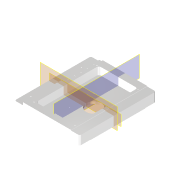
# Autodesk Inventor part: 00_xystage_gp-010b_base
Saved by Autodesk Inventor 2022 (Build 260153000, 153)
## iProperties
Created: 2022-06-02
Part Number: 00_xystage_gp-010b_base
Material: Generisch
Document SubType Name: Modellieren
Designer: diederichbenedict
Density: 1 g/cm^3
Appearance: Glatt - Weiß
Sheet Metal Rule: Standard_mm
Author: diederichbenedict
Autodesk Inventor part; units mm, degrees
ref_plane "YZ Plane" through (0, 0, 0) normal (1, 0, 0) x (0, 1, 0)
ref_plane "XZ Plane" through (0, 0, 0) normal (0, 1, 0) x (-1, 0, 0)
ref_plane "XY Plane" through (0, 0, 0) normal (0, 0, 1) x (1, 0, 0)
sketch "Skizze1" plane through (0, 0, 0) normal (0, 1, 0) x (-1, 0, 0)
  line L0 (76, -93.75) -> (-76, -93.75)
  line L1 (-80, -89.75) -> (-80, 89.75)
  line L2 (-76, 93.75) -> (76, 93.75)
  line L3 (80, 89.75) -> (80, -89.75)
  line L4 (80, -93.75) -> (-80, 93.75) construction
  line L5 (-80, -93.75) -> (80, 93.75) construction
  arc A0 (80, 89.75) -> (76, 93.75) centre (76, 89.75) ccw
  arc A1 (76, -93.75) -> (80, -89.75) centre (76, -89.75) ccw
  arc A2 (-80, -89.75) -> (-76, -93.75) centre (-76, -89.75) ccw
  arc A3 (-76, 93.75) -> (-80, 89.75) centre (-76, 89.75) ccw
  line L6 (43.7, 77.95) -> (-51.7, 77.95)
  line L7 (-51.7, 77.95) -> (-51.7, -58.6)
  line L8 (-51.7, -58.6) -> (43.7, -58.6)
  line L9 (43.7, -58.6) -> (43.7, 77.95)
  line L10 (43.7, 77.95) -> (-51.7, -58.6) construction
  line L11 (-51.7, 77.95) -> (43.7, -58.6) construction
  point P0 (0, 0)
  point P1 (-4, 9.675)
  dimension "d0" = 160
  dimension "d1" = 187.5
  dimension "d2" = 4
  dimension "d3" = 15.8
  dimension "d4" = 28.3
  dimension "d5" = 35.15
  dimension "d6" = 36.3
  dimension "d32" = 136.55
  dimension "d33" = 95.4
  constraints: 24 end point, 8 point on circle, 8 point on line, 8 tangent, 4 centre point, 4 midpoint, 4 parallel, 3 equal radius, 2 horizontal, 2 perpendicular
  measures "d0" distance of L4.end L5.end
  measures "d1" distance of L5.start L4.end
  measures "d2" radius of A0
  measures "d3" distance between parallel lines of L6 L2
  measures "d4" distance between parallel lines of L7 L1
  measures "d5" distance between parallel lines of L0 L8
  measures "d6" distance between parallel lines of L3 L9
  measures "d32" distance between parallel lines of L6 L8
  measures "d33" distance between parallel lines of L9 L7
extrude "Extrusion1" add sketch "Skizze1" along normal blind 23.4
sketch "Skizze2" plane through (0, 0, 0) normal (0, -1, 0) x (1, 0, 0)
  line L0 (-76, 93.75) -> (76, 93.75) projected
  arc A0 (-76, 93.75) -> (-80, 89.75) centre (-76, 89.75) ccw projected
  line L1 (-80, -89.75) -> (-80, 89.75) projected
  arc A1 (-80, -89.75) -> (-76, -93.75) centre (-76, -89.75) ccw projected
  line L2 (76, -93.75) -> (-76, -93.75) projected
  arc A2 (76, -93.75) -> (80, -89.75) centre (76, -89.75) ccw projected
  line L3 (80, 89.75) -> (80, -89.75) projected
  arc A3 (80, 89.75) -> (76, 93.75) centre (76, 89.75) ccw projected
  line L4 (-43.7, 77.95) -> (-43.7, -58.6) projected
  line L5 (51.7, 77.95) -> (-43.7, 77.95) projected
  line L6 (51.7, -58.6) -> (51.7, 77.95) projected
  line L7 (-43.7, -58.6) -> (51.7, -58.6) projected
  circle A4 centre (20.7, -0.35) radius 18.75
  point P0 (0, 0)
  dimension "d9" = 37.5
  dimension "d11" = 94.1
  dimension "d14" = 59.3
  constraints: 1 centre point
  measures "d9" diameter of A4
  measures "d11" distance from line of L0 A4.centre
  measures "d14" distance from line of L3 A4.centre
extrude "Extrusion2" add sketch "Skizze2" against normal blind 5 contours L0 A3 L3 A2 L2 A1 L1 A0 | L5 L6 L7 L4
sketch "Skizze3" plane through (-76, 23.4, 93.75) normal (0, 1, 0) x (1, 0, 0)
  line L0 (0, 0) -> (152, 0) projected
  arc A0 (152, 0) -> (156, 4) centre (152, 4) ccw projected
  line L1 (156, 4) -> (156, 183.5) projected
  arc A1 (156, 183.5) -> (152, 187.5) centre (152, 183.5) ccw projected
  line L2 (152, 187.5) -> (0, 187.5) projected
  arc A2 (0, 187.5) -> (-4, 183.5) centre (0, 183.5) ccw projected
  line L3 (-4, 183.5) -> (-4, 4) projected
  arc A3 (-4, 4) -> (0, 0) centre (0, 4) ccw projected
  line L4 (32.3, 15.8) -> (32.3, 152.35) projected
  line L5 (32.3, 152.35) -> (127.7, 152.35) projected
  line L6 (127.7, 152.35) -> (127.7, 15.8) projected
  line L7 (127.7, 15.8) -> (32.3, 15.8) projected
  line L8 (152, 187.5) -> (0, 187.5) projected
  line L9 (-4, 0) -> (16.8, 0)
  line L10 (16.8, 0) -> (16.8, 187.5)
  line L11 (16.8, 187.5) -> (-4, 187.5)
  line L12 (-4, 187.5) -> (-4, 0)
  point P0 (76, 93.75)
  dimension "d69" = 20.8
  constraints: 8 end point, 2 parallel, 1 horizontal, 1 perpendicular, 1 point on line
  measures "d69" distance of L11.end L10.end
extrude "Extrusion3" cut sketch "Skizze3" against normal blind 6.5 contours A3 L3 A2 L2 L10 L0
ref_plane "Arbeitsebene1" through (4, 23.4, -58.6) normal (-1, 0, 0) x (0, 0, 1)
ref_plane "Arbeitsebene2" through (-43.7, 23.4, 9.675) normal (0, 0, 1) x (1, 0, 0)
fillet "Rundung1" radius 6 4 edges at (-43.7, 14.2, -58.6) (-43.7, 14.2, 77.95) (51.7, 14.2, 77.95) (51.7, 14.2, -58.6)
sketch "Skizze8" plane through (0, 0, 0) normal (0, -1, 0) x (1, 0, 0)
  circle A0 centre (20.7, -0.35) radius 18.75 projected
  line L0 (-9.3, 29.65) -> (50.7, 29.65)
  line L1 (50.7, 29.65) -> (50.7, -30.35)
  line L2 (50.7, -30.35) -> (-9.3, -30.35)
  line L3 (-9.3, -30.35) -> (-9.3, 29.65)
  line L4 (-9.3, 29.65) -> (50.7, -30.35) construction
  line L5 (50.7, 29.65) -> (-9.3, -30.35) construction
  circle A1 centre (50.7, -30.35) radius 1.25
  circle A2 centre (-9.3, -30.35) radius 1.25
  circle A3 centre (-9.3, 29.65) radius 1.25
  circle A4 centre (50.7, 29.65) radius 1.25
  point P0 (0, 0)
  dimension "d61" = 60
  dimension "d62" = 60
  dimension "d63" = 2.5
  dimension "d64" = 2.5
  dimension "d65" = 2.5
  dimension "d66" = 2.5
  constraints: 12 end point, 4 centre point, 4 coincident, 2 midpoint, 2 parallel, 1 horizontal, 1 perpendicular
  measures "d61" distance of L1.end L2.end
  measures "d62" distance of L0.end L1.end
  measures "d63" diameter of A1
  measures "d64" diameter of A2
  measures "d65" diameter of A3
  measures "d66" diameter of A4
extrude "Extrusion6" cut sketch "Skizze8" against normal blind 10 contours L3 A3 L0 | L0 A3 L3 | A4 L1 L0 | L0 L1 A4 | A2 L2 L3 | L3 L2 A2 | A1 L2 L1 | L1 L2 A1
sketch "Skizze9" plane through (0, 23.4, 0) normal (0, 1, 0) x (1, 0, 0)
  line L0 (-59.2, 93.75) -> (-59.2, -93.75) projected
  line L1 (-59.2, -93.75) -> (76, -93.75) projected
  arc A0 (76, -93.75) -> (80, -89.75) centre (76, -89.75) ccw projected
  line L2 (80, -89.75) -> (80, 89.75) projected
  arc A1 (80, 89.75) -> (76, 93.75) centre (76, 89.75) ccw projected
  line L3 (76, 93.75) -> (-59.2, 93.75) projected
  line L4 (-43.7, -71.95) -> (-43.7, 52.6) projected
  arc A2 (-37.7, 58.6) -> (-43.7, 52.6) centre (-37.7, 52.6) ccw projected
  line L5 (-37.7, 58.6) -> (45.7, 58.6) projected
  arc A3 (51.7, 52.6) -> (45.7, 58.6) centre (45.7, 52.6) ccw projected
  line L6 (51.7, 52.6) -> (51.7, -71.95) projected
  arc A4 (45.7, -77.95) -> (51.7, -71.95) centre (45.7, -71.95) ccw projected
  line L7 (45.7, -77.95) -> (-37.7, -77.95) projected
  arc A5 (-43.7, -71.95) -> (-37.7, -77.95) centre (-37.7, -71.95) ccw projected
  line L8 (80, 93.75) -> (58.8, 93.75)
  line L9 (58.8, 93.75) -> (58.8, -93.75)
  line L10 (58.8, -93.75) -> (80, -93.75)
  line L11 (80, -93.75) -> (80, 93.75)
  point P0 (0, 0)
  dimension "d70" = 21.2
  constraints: 8 end point, 2 parallel, 1 horizontal, 1 perpendicular, 1 point on line
  measures "d70" distance between parallel lines of L9 L2
extrude "Extrusion7" cut sketch "Skizze9" against normal blind 1.3 contours L3 A1 L2 A0 L1 L9
sketch "Skizze10" plane through (0, 23.4, 0) normal (0, 1, 0) x (1, 0, 0)
  line L0 (58.8, -93.75) -> (58.8, 93.75) projected
  line L1 (58.8, 93.75) -> (-59.2, 93.75) projected
  line L2 (-59.2, 93.75) -> (-59.2, -93.75) projected
  line L3 (-59.2, -93.75) -> (58.8, -93.75) projected
  line L4 (-43.7, -71.95) -> (-43.7, 52.6) projected
  arc A0 (-37.7, 58.6) -> (-43.7, 52.6) centre (-37.7, 52.6) ccw projected
  line L5 (-37.7, 58.6) -> (45.7, 58.6) projected
  arc A1 (51.7, 52.6) -> (45.7, 58.6) centre (45.7, 52.6) ccw projected
  line L6 (51.7, 52.6) -> (51.7, -71.95) projected
  arc A2 (45.7, -77.95) -> (51.7, -71.95) centre (45.7, -71.95) ccw projected
  line L7 (45.7, -77.95) -> (-37.7, -77.95) projected
  arc A3 (-43.7, -71.95) -> (-37.7, -77.95) centre (-37.7, -71.95) ccw projected
  line L8 (-59.2, 93.75) -> (-59.2, -93.75) projected
  line L9 (-59.2, 93.75) -> (-50.6, 93.75)
  line L10 (-50.6, 93.75) -> (-50.6, 2.35)
  line L11 (-50.6, 2.35) -> (-59.2, 2.35)
  line L12 (-59.2, 2.35) -> (-59.2, 93.75)
  point P0 (0, 0)
  dimension "d73" = 8.6
  dimension "d74" = 91.4
  constraints: 8 end point, 2 parallel, 1 horizontal, 1 perpendicular
  measures "d73" distance of L10.end L11.end
  measures "d74" distance of L9.end L10.end
extrude "Extrusion8" cut sketch "Skizze10" against normal blind 3.3 contours L10 L11 L2 L1
fillet "Rundung2" radius 10 1 edges at (-50.6, 21.75, -2.35)
sketch "Skizze11" plane through (0, 0, 0) normal (0, -1, 0) x (1, 0, 0)
  circle A0 centre (-9.3, 29.65) radius 1.25 projected
  circle A1 centre (-9.3, -30.35) radius 1.25 projected
  circle A2 centre (50.7, 29.65) radius 1.25 projected
  circle A3 centre (50.7, -30.35) radius 1.25 projected
  circle A4 centre (20.7, -0.35) radius 18.75 projected
  line L0 (-76, 93.75) -> (76, 93.75) projected
  arc A5 (-76, 93.75) -> (-80, 89.75) centre (-76, 89.75) ccw projected
  line L1 (-80, -89.75) -> (-80, 89.75) projected
  arc A6 (-80, -89.75) -> (-76, -93.75) centre (-76, -89.75) ccw projected
  line L2 (76, -93.75) -> (-76, -93.75) projected
  arc A7 (76, -93.75) -> (80, -89.75) centre (76, -89.75) ccw projected
  line L3 (80, 89.75) -> (80, -89.75) projected
  arc A8 (80, 89.75) -> (76, 93.75) centre (76, 89.75) ccw projected
  line L4 (-80, 89.75) -> (-80, -89.75) projected
  line L5 (-80, -67.75) -> (80, -67.75)
  line L6 (80, -67.75) -> (80, 67.75)
  line L7 (80, 67.75) -> (-80, 67.75)
  line L8 (-80, 67.75) -> (-80, -67.75)
  point P0 (0, 0)
  point P1 (-80, 67.75)
  dimension "d78" = 26
  dimension "d79" = 26
  constraints: 8 end point, 2 parallel, 2 point on line, 1 horizontal, 1 perpendicular
  measures "d78" distance between parallel lines of L2 L5
  measures "d79" distance between parallel lines of L0 L7
extrude "Extrusion9" add sketch "Skizze11" along normal blind 0.8 contours L7 L3 L5 L1
sketch "Skizze12" plane through (0, 23.4, 0) normal (0, 1, 0) x (1, 0, 0)
  circle A0 centre (-68.5, -66.25) radius 1.4
  circle A1 centre (-68.5, 58.75) radius 1.4
  line L0 (-80, -89.75) -> (-80, 89.75) projected
  line L1 (-76, 93.75) -> (-59.2, 93.75) projected
  line L2 (-43.7, -71.95) -> (-43.7, 52.6) projected
  arc A2 (-37.7, 58.6) -> (-43.7, 52.6) centre (-37.7, 52.6) ccw projected
  line L3 (-37.7, 58.6) -> (45.7, 58.6) projected
  arc A3 (51.7, 52.6) -> (45.7, 58.6) centre (45.7, 52.6) ccw projected
  line L4 (51.7, 52.6) -> (51.7, -71.95) projected
  arc A4 (45.7, -77.95) -> (51.7, -71.95) centre (45.7, -71.95) ccw projected
  line L5 (45.7, -77.95) -> (-37.7, -77.95) projected
  arc A5 (-43.7, -71.95) -> (-37.7, -77.95) centre (-37.7, -71.95) ccw projected
  line L6 (-50.6, 93.75) -> (-50.6, 12.2515) projected
  arc A6 (-59.2, 2.35) -> (-50.6, 12.2515) centre (-60.6, 12.2515) ccw projected
  line L7 (-59.2, 2.35) -> (-59.2, -93.75) projected
  line L8 (-59.2, -93.75) -> (58.8, -93.75) projected
  line L9 (58.8, -93.75) -> (58.8, 93.75) projected
  line L10 (58.8, 93.75) -> (-50.6, 93.75) projected
  line L11 (45.7, 64.6) -> (-37.7, 64.6)
  arc A7 (-37.7, 64.6) -> (-49.7, 52.6) centre (-37.7, 52.6) ccw
  line L12 (-49.7, 52.6) -> (-49.7, -71.95)
  arc A8 (-49.7, -71.95) -> (-37.7, -83.95) centre (-37.7, -71.95) ccw
  line L13 (-37.7, -83.95) -> (45.7, -83.95)
  arc A9 (45.7, -83.95) -> (57.7, -71.95) centre (45.7, -71.95) ccw
  line L14 (57.7, -71.95) -> (57.7, 52.6)
  arc A10 (57.7, 52.6) -> (45.7, 64.6) centre (45.7, 52.6) ccw
  line L15 (-46.1853, 61.0853) -> (54.1853, -80.4353)
  line L16 (54.1853, 61.0853) -> (-46.1853, -80.4353)
  circle A11 centre (-46.1853, 61.0853) radius 1.4
  circle A12 centre (54.1853, 61.0853) radius 1.4
  circle A13 centre (54.1853, -80.4353) radius 1.4
  circle A14 centre (-46.1853, -80.4353) radius 1.4
  line L17 (-46.1853, -80.4353) -> (54.1853, -80.4353)
  line L18 (54.1853, -80.4353) -> (54.1853, 74.5647)
  line L19 (54.1853, 74.5647) -> (-46.1853, 74.5647)
  line L20 (-46.1853, 74.5647) -> (-46.1853, -80.4353)
  circle A15 centre (54.1853, 74.5647) radius 1.4
  circle A16 centre (-46.1853, 74.5647) radius 1.4
  point P0 (0, 0)
  dimension "d82" = 2.8
  dimension "d83" = 2.8
  dimension "d84" = 11.5
  dimension "d85" = 11.5
  dimension "d86" = 35
  dimension "d87" = 125
  dimension "d90" = 6
  dimension "d91" = 2.8
  dimension "d92" = 2.8
  dimension "d93" = 2.8
  dimension "d94" = 2.8
  dimension "d151" = 155
  dimension "d152" = 2.8
  dimension "d153" = 2.8
  constraints: 20 end point, 12 centre point, 12 point on circle, 10 coincident, 2 parallel, 1 horizontal, 1 perpendicular, 7 other
  measures "d82" diameter of A0
  measures "d83" diameter of A1
  measures "d84" distance from line of A1.centre L0
  measures "d85" distance from line of A0.centre L0
  measures "d86" distance from line of A1.centre L1
  measures "d87" distance of A1.centre A0.centre
  measures "d90" distance between parallel lines of L3 L11
  measures "d91" diameter of A11
  measures "d92" diameter of A12
  measures "d93" diameter of A13
  measures "d94" diameter of A14
  measures "d151" distance of L18.end L17.end
  measures "d152" diameter of A15
  measures "d153" diameter of A16
extrude "Extrusion10" cut sketch "Skizze12" along normal mid plane 2 contours A0 | A1 | A14 L17 L16 | L16 L20 A14 | A8 A14 | L17 A14 A8 | A8 A14 L20 | A13 L18 L15 | L15 L17 A13 | L17 A9 A13 | A9 A13 | L18 A13 A9 | A16 L19 L20 | L20 L19 A16 | A15 L19 L18 | L18 L19 A15
sketch "Skizze13" plane through (0, 0, 0) normal (0, -1, 0) x (1, 0, 0)
  line L0 (80, -67.75) -> (-80, -67.75) projected
  line L1 (-80, -89.75) -> (-80, -67.75) projected
  arc A0 (-80, -89.75) -> (-76, -93.75) centre (-76, -89.75) ccw projected
  line L2 (76, -93.75) -> (-76, -93.75) projected
  arc A1 (76, -93.75) -> (80, -89.75) centre (76, -89.75) ccw projected
  line L3 (80, -67.75) -> (80, -89.75) projected
  circle A2 centre (-50, -77.75) radius 1.6
  circle A3 centre (44.9947, -76.75) radius 1.6
  line L4 (-80, 67.75) -> (-80, -67.75) projected
  line L5 (-80, -67.75) -> (80, -67.75) projected
  line L6 (80, -67.75) -> (80, 67.75) projected
  line L7 (80, 67.75) -> (-80, 67.75) projected
  circle A4 centre (20.7, -0.35) radius 18.75 projected
  circle A5 centre (-9.3, 29.65) radius 1.25 projected
  circle A6 centre (-9.3, -30.35) radius 1.25 projected
  circle A7 centre (50.7, 29.65) radius 1.25 projected
  circle A8 centre (50.7, -30.35) radius 1.25 projected
  circle A9 centre (-32.2212, -61.75) radius 1.6
  circle A10 centre (-16.2212, -61.75) radius 1.6
  circle A11 centre (-0.2212, -61.75) radius 1.6
  circle A12 centre (15.7788, -61.75) radius 1.4
  circle A13 centre (31.7788, -61.75) radius 1.4
  point P0 (0, 0)
  dimension "d95" = 3.2
  dimension "d96" = 3.2
  dimension "d97" = 30
  dimension "d98" = 95
  dimension "d99" = 16
  dimension "d100" = 17
  dimension "d101" = 3.2
  dimension "d102" = 3.2
  dimension "d103" = 3.2
  dimension "d104" = 16
  dimension "d105" = 0
  dimension "d106" = 0
  dimension "d107" = 16
  dimension "d108" = 16
  dimension "d134" = 2.8
  dimension "d135" = 2.8
  dimension "d136" = 16
  dimension "d137" = 16
  constraints: 7 centre point
  measures "d95" diameter of A2
  measures "d96" diameter of A3
  measures "d97" distance from line of A2.centre L1
  measures "d98" distance of A3.centre A2.centre
  measures "d99" distance from line of A2.centre L2
  measures "d100" distance from line of A3.centre L2
  measures "d101" diameter of A9
  measures "d102" diameter of A10
  measures "d103" diameter of A11
  measures "d104" vertical distance of A9.centre A2.centre
  measures "d105" vertical distance of A9.centre A10.centre
  measures "d106" vertical distance of A10.centre A11.centre
  measures "d107" distance of A10.centre A9.centre
  measures "d108" distance of A11.centre A10.centre
  measures "d134" diameter of A12
  measures "d135" diameter of A13
  measures "d136" distance of A12.centre A13.centre
  measures "d137" distance of A11.centre A12.centre
extrude "Extrusion11" cut sketch "Skizze13" along normal mid plane 2 contours A2 | A3 | A9 | A10 | A11 | A12 | A13
sketch "Skizze14" plane through (0, -0.8, 0) normal (0, -1, 0) x (1, 0, 0)
  line L0 (-80, 67.75) -> (-80, -67.75) projected
  line L1 (-80, -67.75) -> (80, -67.75) projected
  line L2 (80, -67.75) -> (80, 67.75) projected
  line L3 (80, 67.75) -> (-80, 67.75) projected
  circle A0 centre (20.7, -0.35) radius 18.75 projected
  circle A1 centre (-9.3, 29.65) radius 1.25 projected
  circle A2 centre (-9.3, -30.35) radius 1.25 projected
  circle A3 centre (50.7, 29.65) radius 1.25 projected
  circle A4 centre (50.7, -30.35) radius 1.25 projected
  line L4 (-0.3, 20.65) -> (41.7, 20.65) construction
  line L5 (41.7, 20.65) -> (41.7, -21.35) construction
  line L6 (41.7, -21.35) -> (-0.3, -21.35) construction
  line L7 (-0.3, -21.35) -> (-0.3, 20.65) construction
  line L8 (-0.3, 20.65) -> (41.7, -21.35) construction
  line L9 (41.7, 20.65) -> (-0.3, -21.35) construction
  point P0 (0, 0)
  dimension "d111" = 42
  dimension "d112" = 42
  constraints: 12 end point, 2 midpoint, 2 parallel, 1 horizontal, 1 perpendicular
  measures "d111" distance of L5.end L6.end
  measures "d112" distance of L4.end L5.end
hole "Bohrung3" at (-0.3, -0.8, 20.65) at (41.7, -0.8, 20.65) at (41.7, -0.8, -21.35) at (-0.3, -0.8, -21.35) direction (0, 1, 0) diameter 2.8 depth 1 tip angle 118
pattern_linear "Rechteckige Anordnung1" count 3 spacing 50 along (-1, 0, 0) count 3 spacing 50 along (0, 0, 1) of "Bohrung3" first direction both ways yes second direction both ways yes
sketch "Skizze15" plane through (0, 23.4, 0) normal (0, 1, 0) x (1, 0, 0)
  line L0 (-43.7, -71.95) -> (-43.7, 52.6) projected
  arc A0 (-37.7, 58.6) -> (-43.7, 52.6) centre (-37.7, 52.6) ccw projected
  line L1 (-37.7, 58.6) -> (45.7, 58.6) projected
  arc A1 (51.7, 52.6) -> (45.7, 58.6) centre (45.7, 52.6) ccw projected
  line L2 (51.7, 52.6) -> (51.7, -71.95) projected
  arc A2 (45.7, -77.95) -> (51.7, -71.95) centre (45.7, -71.95) ccw projected
  line L3 (45.7, -77.95) -> (-37.7, -77.95) projected
  arc A3 (-43.7, -71.95) -> (-37.7, -77.95) centre (-37.7, -71.95) ccw projected
  line L4 (-50.6, 93.75) -> (-50.6, 12.2515) projected
  arc A4 (-59.2, 2.35) -> (-50.6, 12.2515) centre (-60.6, 12.2515) ccw projected
  line L5 (-59.2, 2.35) -> (-59.2, -93.75) projected
  line L6 (-59.2, -93.75) -> (58.8, -93.75) projected
  line L7 (58.8, -93.75) -> (58.8, 93.75) projected
  line L8 (58.8, 93.75) -> (-50.6, 93.75) projected
  line L9 (-43.7, -77.95) -> (51.7, -77.95)
  line L10 (51.7, -77.95) -> (51.7, 72.05)
  line L11 (46.7, 77.05) -> (-38.7, 77.05)
  line L12 (-43.7, 72.05) -> (-43.7, -77.95)
  arc A5 (-38.7, 77.05) -> (-43.7, 72.05) centre (-38.7, 72.05) ccw
  arc A6 (51.7, 72.05) -> (46.7, 77.05) centre (46.7, 72.05) ccw
  circle A7 centre (-46.1853, 74.5647) radius 1.4
  circle A8 centre (54.1853, 74.5647) radius 1.4
  point P0 (0, 0)
  point P1 (51.7, 77.05)
  dimension "d126" = 155
  dimension "d127" = 5
  dimension "d130" = 2.8
  dimension "d131" = 2.8
  constraints: 8 end point, 4 centre point, 4 point on circle, 4 tangent, 2 parallel, 2 point on line, 1 equal radius, 1 horizontal, 1 perpendicular
  measures "d126" distance of point (51.7, 77.05) L9.end
  measures "d127" radius of A5
  measures "d130" diameter of A7
  measures "d131" diameter of A8
extrude "Extrusion12" cut sketch "Skizze15" against normal up to surface (18.4 mm away) contours L0 A0 L1 A1 L2 A2 L3 A3 | L12 A5 L11 A6 L10 A1 L1 A0
sketch "Skizze16" plane through (0, 23.4, 0) normal (0, 1, 0) x (1, 0, 0)
  arc A0 (-59.2, 2.35) -> (-50.6, 12.2515) centre (-60.6, 12.2515) ccw projected
  line L0 (-50.6, 93.75) -> (-50.6, 12.2515) projected
  line L1 (-59.2, 93.75) -> (-50.6, 93.75) projected
  line L2 (-59.2, 2.35) -> (-59.2, 93.75) projected
  circle A1 centre (-54.9, 12.2515) radius 1.4
  circle A2 centre (-54.9, 28.2515) radius 1.4
  circle A3 centre (-54.9, 44.2515) radius 1.4
  circle A4 centre (-54.9, 60.2515) radius 1.4
  circle A5 centre (-54.9, 76.2515) radius 1.4
  point P0 (0, 0)
  dimension "d138" = 2.8
  dimension "d139" = 2.8
  dimension "d140" = 2.8
  dimension "d141" = 2.8
  dimension "d142" = 16
  dimension "d143" = 16
  dimension "d144" = 16
  dimension "d145" = 2.8
  dimension "d146" = 16
  constraints: 5 centre point
  measures "d138" diameter of A1
  measures "d139" diameter of A2
  measures "d140" diameter of A3
  measures "d141" diameter of A4
  measures "d142" distance of A2.centre A1.centre
  measures "d143" distance of A3.centre A2.centre
  measures "d144" distance of A4.centre A3.centre
  measures "d145" diameter of A5
  measures "d146" distance of A5.centre A4.centre
extrude "Extrusion13" cut sketch "Skizze16" against normal blind 4 contours A1 | A2 | A3 | A4 | A5
sketch "Skizze18" plane through (-76, 16.9, 93.75) normal (0, 1, 0) x (1, 0, 0)
  line L0 (-4, 4) -> (-4, 183.5) projected
  line L1 (0, 187.5) -> (16.8, 187.5) projected
  point P0 (76, 93.75)
  point P1 (7.5, 27.5)
  point P2 (7.5, 152.5)
  dimension "d161" = 11.5
  dimension "d162" = 11.5
  dimension "d163" = 125
  dimension "d164" = 35
  measures "d161" distance from line of point (7.5, 27.5) L0
  measures "d162" distance from line of point (7.5, 152.5) L0
  measures "d163" distance of point (7.5, 152.5) point (7.5, 27.5)
  measures "d164" distance from line of L1 point (7.5, 152.5)
hole "Bohrung4" at (-68.5, 16.9, -58.75) at (-68.5, 16.9, 66.25) direction (0, -1, 0) diameter 2.9 depth 1 tip angle 118
sketch "Skizze19" plane through (0, -0.8, 0) normal (0, -1, 0) x (1, 0, 0)
  arc A0 (-9.6873, 28.4615) -> (-8.1115, 30.0373) centre (-8.3, 28.65) ccw projected
  arc A1 (-8.1115, 30.0373) -> (-9.6873, 28.4615) centre (-9.3, 29.65) ccw projected
  arc A2 (49.5115, 30.0373) -> (51.0873, 28.4615) centre (49.7, 28.65) ccw projected
  arc A3 (51.0873, 28.4615) -> (49.5115, 30.0373) centre (50.7, 29.65) ccw projected
  arc A4 (-8.1115, -30.7373) -> (-9.6873, -29.1615) centre (-8.3, -29.35) ccw projected
  arc A5 (-9.6873, -29.1615) -> (-8.1115, -30.7373) centre (-9.3, -30.35) ccw projected
  arc A6 (51.0873, -29.1615) -> (49.5115, -30.7373) centre (49.7, -29.35) ccw projected
  arc A7 (49.5115, -30.7373) -> (51.0873, -29.1615) centre (50.7, -30.35) ccw projected
  circle A8 centre (-50.3, 28.65) radius 1.4 projected
  circle A9 centre (41.7, 28.65) radius 1.4 projected
  circle A10 centre (-0.3, 28.65) radius 1.4 projected
  circle A11 centre (-8.3, -21.35) radius 1.4 projected
  circle A12 centre (-50.3, 20.65) radius 1.4 projected
  circle A13 centre (-8.3, 20.65) radius 1.4 projected
  circle A14 centre (-50.3, -21.35) radius 1.4 projected
  circle A15 centre (49.7, 20.65) radius 1.4 projected
  circle A16 centre (49.7, -21.35) radius 1.4 projected
  circle A17 centre (-50.3, -29.35) radius 1.4 projected
  circle A18 centre (-0.3, -29.35) radius 1.4 projected
  circle A19 centre (41.7, -29.35) radius 1.4 projected
  circle A20 centre (41.7, -21.35) radius 1.4 projected
  circle A21 centre (-0.3, 20.65) radius 1.4 projected
  circle A22 centre (41.7, 20.65) radius 1.4 projected
  circle A23 centre (-0.3, -21.35) radius 1.4 projected
  circle A24 centre (-0.2212, -61.75) radius 1.6 projected
  circle A25 centre (15.7788, -61.75) radius 1.4 projected
  circle A26 centre (-16.2212, -61.75) radius 1.6 projected
  circle A27 centre (-32.2212, -61.75) radius 1.6 projected
  circle A28 centre (31.7788, -61.75) radius 1.4 projected
  line L0 (-80, 67.75) -> (-80, -67.75) projected
  line L1 (-80, -67.75) -> (80, -67.75) projected
  line L2 (80, -67.75) -> (80, 67.75) projected
  line L3 (80, 67.75) -> (-80, 67.75) projected
  circle A29 centre (20.7, -0.35) radius 18.75 projected
  circle A30 centre (73.2, 44.45) radius 2
  circle A31 centre (73.2, -43.75) radius 2
  line L4 (-59.2, -93.75) -> (-59.2, 93.75) projected
  line L5 (-76, 93.75) -> (76, 93.75) projected
  line L6 (76, -93.75) -> (-76, -93.75) projected
  circle A32 centre (-69.7, 0) radius 2
  circle A33 centre (-69.7, -43.75) radius 2
  circle A34 centre (-69.7, 44.45) radius 2
  circle A35 centre (73.2, 0) radius 2
  point P0 (0, 0)
  dimension "d165" = 6.8
  dimension "d166" = 0
  dimension "d167" = 49.3
  dimension "d168" = 50
  dimension "d169" = 4
  dimension "d170" = 4
  dimension "d171" = 88.2
  dimension "d173" = 10.3
  dimension "d174" = 93.75
  dimension "d175" = 4
  dimension "d182" = 4
  dimension "d183" = 4
  dimension "d184" = 4
  constraints: 6 centre point
  measures "d165" distance from line of A30.centre L2
  measures "d166" horizontal distance of A31.centre A30.centre
  measures "d167" distance from line of L5 A30.centre
  measures "d168" distance from line of L6 A31.centre
  measures "d169" diameter of A30
  measures "d170" diameter of A31
  measures "d171" distance of A30.centre A31.centre
  measures "d173" distance from line of L0 A32.centre
  measures "d174" distance from line of A32.centre L6
  measures "d175" diameter of A32
  measures "d182" diameter of A33
  measures "d183" diameter of A34
  measures "d184" diameter of A35
extrude "Extrusion15" cut sketch "Skizze19" against normal blind 10 contours A30 | A31 | A32
ref_plane "Arbeitsebene3" through (-76, 0, 0) normal (0, 0, 1) x (1, 0, 0)
equation "\"Biegeradius\" = Stärke"
equation "\"BreiteBiegungsfreistellung\" = Stärke"
equation "\"TiefeBiegungsfreistellung\" = 0.5 * Stärke"
equation "\"GrößeEckenfreistellung\" = 4 * Stärke"
equation "\"MinimalRest\" = 2 * Stärke"
equation "\"Übergangsradius\" = Biegeradius"
equation "\"JacobiRadiusGröße\" = Biegeradius"
equation "\"Abstandsgröße\" = Stärke"
equation "\"Stärke\" = 0.5"
